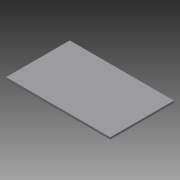
# Autodesk Inventor part: bottom
Saved by Autodesk Inventor 2013 SP1 (Build 170176100, 176)
## iProperties
Created: 2019-01-15
Part Number: bottom
Material: Типовые
Document SubType Name: Modeling
Designer: jhcjhguw
Density: 1 g/cm^3
Author: jhcjhguw
Autodesk Inventor part; units mm, degrees
ref_plane "YZ Plane" through (0, 0, 0) normal (1, 0, 0) x (0, 1, 0)
ref_plane "XZ Plane" through (0, 0, 0) normal (0, 1, 0) x (-1, 0, 0)
ref_plane "XY Plane" through (0, 0, 0) normal (0, 0, 1) x (1, 0, 0)
sketch "Эскиз1" plane through (0, 0, 0) normal (0, 0, 1) x (1, 0, 0)
  line L0 (0, 0) -> (104.8, 0)
  line L1 (104.8, 0) -> (104.8, 64)
  line L2 (104.8, 64) -> (0, 64)
  line L3 (0, 64) -> (0, 0)
  dimension "d0" = 104.8
  dimension "d1" = 64
  constraints: 8 end point, 2 parallel, 1 horizontal, 1 perpendicular
  measures "d0" distance of L2.end L1.end
  measures "d1" distance of L1.end L0.end
extrude "Выдавливание1" add sketch "Эскиз1" along normal blind 2
